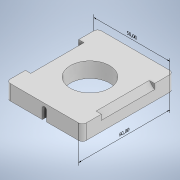
# Autodesk Inventor part: SmartWatch_BaseTop
Saved by Autodesk Inventor 2020.3 (Build 243373000, 373)
## iProperties
Created: 2020-02-20
Part Number: SmartWatch_BaseTop
Material: Generic
Document SubType Name: Modeling
Designer: super
Density: 1 g/cm^3
Appearance: Default
Author: super
Autodesk Inventor part; units mm, degrees
ref_plane "YZ Plane" through (0, 0, 0) normal (1, 0, 0) x (0, 1, 0)
ref_plane "XZ Plane" through (0, 0, 0) normal (0, 1, 0) x (-1, 0, 0)
ref_plane "XY Plane" through (0, 0, 0) normal (0, 0, 1) x (1, 0, 0)
sketch "Sketch1" plane through (0, 0, 0) normal (0, 1, 0) x (-1, 0, 0)
  line L0 (0, 0) -> (50, 0)
  line L1 (50, 0) -> (50, -30)
  line L2 (50, -30) -> (0, -30)
  line L3 (0, -30) -> (0, 0)
  dimension "d0" = 50
  dimension "d1" = 30
  constraints: 8 end point, 2 perpendicular, 1 horizontal, 1 vertical
  measures "d0" distance of L0.start L0.end
  measures "d1" distance of L0.end L1.end
extrude "Extrusion1" add sketch "Sketch1" along normal blind 10
sketch "Sketch2" plane through (0, 0, -30) normal (0, 0, -1) x (-1, 0, 0)
  line L0 (50, 10) -> (0, 10) projected
  line L1 (0, 10) -> (3.5, 10)
  line L2 (3.5, 10) -> (0, 6.5)
  line L3 (0, 0) -> (0, 10) projected
  line L4 (0, 6.5) -> (0, 10)
  constraints: 6 end point, 2 point on line, 1 collinear
extrude "Extrusion2" cut sketch "Sketch2" against normal blind 17.5
sketch "Sketch3" plane through (0, 0, -30) normal (0, 0, -1) x (-1, 0, 0)
  line L0 (50, 0) -> (50, 10) projected
  line L1 (50, 10) -> (50, 6.5)
  line L2 (50, 6.5) -> (46.5, 10)
  line L3 (50, 10) -> (0, 10) projected
  line L4 (46.5, 10) -> (50, 10)
  line L5 (50, 10) -> (50, 6.5)
  point P0 (0, 0)
  constraints: 8 end point, 2 collinear, 2 point on line
extrude "Extrusion3" cut sketch "Sketch3" against normal blind 17.5
sketch "Sketch4" plane through (0, 0, -30) normal (0, 0, -1) x (-1, 0, 0)
  line L0 (0, 0) -> (50, 0) projected
  line L1 (3.5, 10) -> (0, 6.5) projected
  line L2 (0, 0) -> (0, 6.5)
  line L3 (3.5, 10) -> (46.5, 10) projected
  line L4 (0, 6.5) -> (3.5, 10)
  line L5 (3.5, 10) -> (46.5, 10)
  line L6 (46.5, 10) -> (50, 6.5)
  line L7 (50, 0) -> (50, 10) projected
  line L8 (50, 6.5) -> (50, 0)
  line L9 (0, 0) -> (0, 10) projected
  line L10 (50, 0) -> (0, 0)
  constraints: 12 end point, 2 perpendicular, 2 vertical, 1 collinear, 1 point on line
extrude "Extrusion4" add sketch "Sketch4" along normal blind 30
sketch "Sketch5" plane through (0, 0, -60) normal (0, 0, -1) x (-1, 0, 0)
  line L0 (3.5, 10) -> (0, 6.5) projected
  line L1 (0, 6.5) -> (3.5, 10)
  line L2 (0, 6.5) -> (0, 10) projected
  line L3 (3.5, 10) -> (0, 10)
  line L4 (0, 10) -> (0, 6.5)
  point P0 (0, 0)
  constraints: 6 end point, 2 perpendicular, 1 collinear
extrude "Extrusion5" add sketch "Sketch5" against normal blind 12.5
sketch "Sketch6" plane through (0, 0, -60) normal (0, 0, -1) x (-1, 0, 0)
  line L0 (50, 6.5) -> (46.5, 10) projected
  line L1 (46.5, 10) -> (50, 6.5)
  line L2 (46.5, 10) -> (50, 10) projected
  line L3 (50, 6.5) -> (50, 10)
  line L4 (50, 10) -> (46.5, 10)
  point P0 (0, 0)
  constraints: 6 end point, 2 perpendicular, 1 collinear
extrude "Extrusion6" add sketch "Sketch6" against normal blind 12.5
fillet "Fillet1" radius 2.5 2 edges at (0, 5, 0) (-50, 5, 0)
sketch "Sketch7" plane through (0, 10, 0) normal (0, 1, 0) x (1, 0, 0)
  line L0 (0, 12.5) -> (0, 47.5) projected
  circle A0 centre (-25, 30) radius 12.95
  point P0 (0, 0)
  dimension "d21" = 25.9
  constraints: 1 centre point
  measures "d21" diameter of A0
extrude "Extrusion7" cut sketch "Sketch7" against normal blind 10
sketch "Sketch8" plane through (-47.5, 0, 0) normal (0, 0, 1) x (1, 0, 0)
  line L0 (1, 10) -> (-2.5, 10) projected
  line L1 (0, 10) -> (45, 10) projected
  circle A0 centre (22.5, 6.7) radius 1.775
  point P0 (47.5, 0)
  dimension "d26" = 3.55
  constraints: 1 centre point
  measures "d26" diameter of A0
extrude "Extrusion8" cut sketch "Sketch8" against normal blind 20
sketch "Sketch9" plane through (-47.5, 0, 0) normal (0, 0, 1) x (1, 0, 0)
  circle A0 centre (22.5, 6.7) radius 1.775 projected
  circle A1 centre (22.5, 6.7) radius 1.775
  point P0 (47.5, 0)
  constraints: 1 centre point, 1 coincident
extrude "Extrusion9" add sketch "Sketch9" against normal blind 6.05
sketch "Sketch10" plane through (-47.5, 0, 0) normal (0, 0, 1) x (1, 0, 0)
  circle A0 centre (22.5, 6.7) radius 1.775 projected
  circle A1 centre (22.5, 6.7) radius 1.36
  point P0 (47.5, 0)
  dimension "d31" = 2.72
  constraints: 1 centre point, 1 coincident
  measures "d31" diameter of A1
extrude "Extrusion10" cut sketch "Sketch10" against normal blind 6.05 contours A1
sketch "Sketch11" plane through (0, 0, 0) normal (0, -1, 0) x (1, 0, 0)
  line L0 (-23.225, -6.05) -> (-23.225, -17.1722) projected
  line L1 (-23.225, -17.1722) -> (-26.775, -17.1722)
  line L2 (-26.775, -6.05) -> (-26.775, -17.1722) projected
  line L3 (-23.225, -6.05) -> (-26.775, -6.05) projected
  line L4 (-26.775, -6.05) -> (-23.225, -6.05)
  line L5 (-23.225, -6.05) -> (-23.225, -17.1722)
  point P0 (0, 0)
  constraints: 6 end point, 2 horizontal, 2 point on line, 1 perpendicular
extrude "Extrusion11" cut sketch "Sketch11" against normal blind 6.7
sketch "Sketch12" plane through (0, 0, 0) normal (0, -1, 0) x (1, 0, 0)
  line L0 (-26.36, 0) -> (-26.36, -6.05) projected
  line L1 (-26.36, 0) -> (-23.64, 0)
  line L2 (-23.64, 0) -> (-23.64, -6.05) projected
  line L3 (-23.64, -6.05) -> (-26.36, -6.05)
  line L4 (-26.36, 0) -> (-23.64, 0) projected
  line L5 (-26.36, -6.05) -> (-26.36, 0)
  point P0 (0, 0)
  constraints: 6 end point, 3 point on line, 2 horizontal, 1 perpendicular
extrude "Extrusion12" cut sketch "Sketch12" against normal blind 6.7
body "Solid1"
